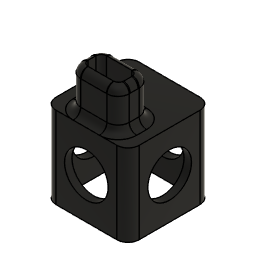
USB C Charger Protector v7 (Autodesk Fusion 360 design; units mm, degrees)
Autodesk Fusion 360 part; units mm, degrees
sketch "Sketch1" plane through (0, 0, 0) normal (0, 0, 1) x (1, 0, 0)
  line L0 (0, 0) -> (-27.6, 0)
  line L1 (-27.6, 0) -> (-27.6, 27.6)
  line L2 (-27.6, 27.6) -> (0, 27.6)
  line L3 (0, 27.6) -> (0, 0)
  line L4 (-27.6, 30.6) -> (-30.6, 30.6)
  line L5 (-30.6, 30.6) -> (3, 30.6)
  line L6 (3, 30.6) -> (3, -3)
  line L7 (3, -3) -> (-30.6, -3)
  line L8 (-30.6, -3) -> (-30.6, 30.6)
  dimension "d1" = 27.6
  dimension "d2" = 27.6
  dimension "d4" = 3
  dimension "d5" = 3
  dimension "d6" = 33.6
  dimension "d7" = 33.6
  constraint horizontal L0
  constraint vertical L1
  constraint horizontal L2
  constraint vertical L3
  constraint coincident L0.start L3.end
  constraint horizontal L5
  constraint vertical L6
  constraint horizontal L7
  constraint vertical L8
  measures "d1" distance of L0.start L0.end
  measures "d2" distance of L0.start L2.end
  measures "d4" distance of L1.end L4.start
  measures "d5" distance of L4.start L4.end
  measures "d6" distance of L4.end L5.end
  measures "d7" distance of L4.end L7.end
extrude "Extrude1" add sketch "Sketch1" along normal blind 30 makes body 1
sketch "Sketch2" plane through (0, 0, 30) normal (0, 0, 1) x (-1, 0, 0)
  line L0 (27.6, -27.6) -> (0, -27.6)
  line L1 (0, -27.6) -> (0, 0)
  line L2 (0, 0) -> (27.6, 0)
  line L3 (27.6, 0) -> (27.6, -27.6)
  line L4 (30.6, 3) -> (-3, 3)
  line L5 (-3, 3) -> (-3, -30.6)
  line L6 (-3, -30.6) -> (30.6, -30.6)
  line L7 (30.6, -30.6) -> (30.6, 3)
  line L8 (30.6, -30.6) -> (-3, -30.6)
  line L9 (-3, -30.6) -> (-3, 3)
  line L10 (-3, 3) -> (30.6, 3)
  line L11 (30.6, 3) -> (30.6, -30.6)
  constraint horizontal L8
  constraint vertical L9
  constraint horizontal L10
  constraint vertical L11
  constraint coincident L4.end L5.start
  constraint coincident L6.end L7.start
extrude "Extrude2" add sketch "Sketch2" along normal blind 3 contours L0 L1 L2 L3 | L4 L5 L6 L7 L8 L9 L10 L11 bodies 1
sketch "Sketch3" plane through (0, 0, 33) normal (0, 0, 1) x (-1, 0, 0)
  line L0 (30.6, 3) -> (-3, 3)
  line L1 (-3, 3) -> (-3, -30.6)
  line L2 (-3, -30.6) -> (30.6, -30.6)
  line L3 (30.6, -30.6) -> (30.6, 3)
  line L4 (18.9169, -2.769) -> (8.6831, -2.769)
  line L5 (6.5511, -4.901) -> (6.5511, -8.099)
  line L6 (8.6831, -10.231) -> (18.9169, -10.231)
  line L7 (21.0489, -8.099) -> (21.0489, -4.901)
  arc A0 (21.0489, -4.901) -> (18.9169, -2.769) centre (18.9169, -4.901) ccw
  arc A1 (18.9169, -10.231) -> (21.0489, -8.099) centre (18.9169, -8.099) ccw
  arc A2 (6.5511, -8.099) -> (8.6831, -10.231) centre (8.6831, -8.099) ccw
  arc A3 (8.6831, -2.769) -> (6.5511, -4.901) centre (8.6831, -4.901) ccw
  line L8 (19.1, -13) -> (8.5, -13)
  line L9 (4, -8.5) -> (4, -4.5)
  line L10 (8.5, 0) -> (19.1, 0)
  line L11 (23.6, -4.5) -> (23.6, -8.5)
  arc A4 (19.1, -13) -> (23.6, -8.5) centre (19.1, -8.5) ccw
  arc A5 (4, -8.5) -> (8.5, -13) centre (8.5, -8.5) ccw
  arc A6 (8.5, 0) -> (4, -4.5) centre (8.5, -4.5) ccw
  arc A7 (23.6, -4.5) -> (19.1, 0) centre (19.1, -4.5) ccw
  point P0 (21.0489, -2.769)
  point P1 (21.0489, -10.231)
  point P2 (23.6, -13)
  point P3 (4, 0)
  point P4 (13.8, -6.5)
  dimension "d62" = 4.5
  constraint vertical L5
  constraint vertical L7
  constraint coincident P0 L4
  constraint coincident P0 L7
  constraint coincident P1 L6
  constraint coincident P1 L7
  constraint horizontal L8
  constraint vertical L9
  constraint horizontal L10
  constraint vertical L11
  constraint tangent L8 A4
  constraint tangent L11 A4
  constraint tangent L8 A5
  constraint tangent L9 A5
  constraint equal A4 A5
  constraint tangent L9 A6
  constraint tangent L10 A6
  constraint equal A4 A6
  constraint tangent L10 A7
  constraint tangent L11 A7
  constraint equal A4 A7
  measures "d62" radius of A4
extrude "Extrude10" add sketch "Sketch3" along normal blind 16 contours L8 L9 L10 L11 A4 A5 A6 A7 bodies 1
fillet "Fillet1" radius 3 4 edges at (-27.6, 27.6, 15) (0, 27.6, 15) (0, 0, 15) (-27.6, 0, 15) on bodies 1
fillet "Fillet2" radius 4.5 4 edges at (3, -3, 16.5) (-30.6, -3, 16.5) (3, 30.6, 16.5) (-30.6, 30.6, 16.5) on bodies 1
sketch "Sketch4" plane through (-30.6, 0, 0) normal (-1, 0, 0) x (0, -1, 0)
  line L0 (-26.1, 33) -> (-26.1, 0)
  line L1 (-26.1, 0) -> (-1.5, 0)
  line L2 (-1.5, 0) -> (-1.5, 33)
  line L3 (-1.5, 33) -> (-26.1, 33)
  circle A0 centre (-13.8, 16.5) radius 8.8142
extrude "Extrude5" cut sketch "Sketch4" against normal blind 33.6 contours A0 bodies 1
sketch "Sketch5" plane through (0, -3, 0) normal (0, -1, 0) x (1, 0, 0)
  line L0 (-26.1, 33) -> (-26.1, 0)
  line L1 (-26.1, 0) -> (-1.5, 0)
  line L2 (-1.5, 0) -> (-1.5, 33)
  line L3 (-1.5, 33) -> (-26.1, 33)
  circle A0 centre (-13.8, 16.5) radius 8.8142
extrude "Extrude6" cut sketch "Sketch5" against normal blind 33.6 contours A0 bodies 1
sketch "Sketch6" plane through (0, 0, 0) normal (0, 0, 1) x (1, 0, 0)
  line L0 (-23.7662, 27.4159) -> (-3.7397, 27.4159)
  line L1 (-0.2397, 23.9159) -> (-0.2397, 3.7722)
  line L2 (-3.7397, 0.2722) -> (-23.7662, 0.2722)
  line L3 (-27.2662, 3.7722) -> (-27.2662, 23.9159)
  arc A0 (-3.7397, 0.2722) -> (-0.2397, 3.7722) centre (-3.7397, 3.7722) ccw
  arc A1 (-27.2662, 3.7722) -> (-23.7662, 0.2722) centre (-23.7662, 3.7722) ccw
  arc A2 (-23.7662, 27.4159) -> (-27.2662, 23.9159) centre (-23.7662, 23.9159) ccw
  arc A3 (-0.2397, 23.9159) -> (-3.7397, 27.4159) centre (-3.7397, 23.9159) ccw
  dimension "d36" = 3.5
  constraint horizontal L0
  constraint vertical L1
  constraint horizontal L2
  constraint vertical L3
  constraint tangent L1 A0
  constraint tangent L2 A0
  constraint tangent L2 A1
  constraint tangent L3 A1
  constraint equal A0 A1
  constraint tangent L0 A2
  constraint tangent L3 A2
  constraint equal A0 A2
  constraint tangent L0 A3
  constraint tangent L1 A3
  constraint equal A0 A3
  measures "d36" radius of A0
extrude "Extrude7" add sketch "Sketch6" along normal blind 29 separate body makes body 2
sketch "Sketch7" plane through (0, 0, 29) normal (0, 0, 1) x (-1, 0, 0)
  arc A0 (3.7397, -0.2722) -> (0.2397, -3.7722) centre (3.7397, -3.7722) ccw
  line L0 (0.2397, -3.7722) -> (0.2397, -23.9159)
  arc A1 (0.2397, -23.9159) -> (3.7397, -27.4159) centre (3.7397, -23.9159) ccw
  line L1 (3.7397, -27.4159) -> (23.7662, -27.4159)
  arc A2 (23.7662, -27.4159) -> (27.2662, -23.9159) centre (23.7662, -23.9159) ccw
  line L2 (27.2662, -23.9159) -> (27.2662, -3.7722)
  arc A3 (27.2662, -3.7722) -> (23.7662, -0.2722) centre (23.7662, -3.7722) ccw
  line L3 (23.7662, -0.2722) -> (3.7397, -0.2722)
  line L4 (18.3436, -8.89) -> (8.1175, -8.89)
  line L5 (8.1175, -4) -> (18.3287, -4)
  arc A4 (18.258, -8.89) -> (18.258, -4) centre (18.3436, -6.445) ccw
  arc A5 (8.1175, -4) -> (8.1175, -8.89) centre (8.1175, -6.445) ccw
  constraint horizontal L4
  constraint coincident L5 A4.end
  constraint coincident L4 A4.start
extrude "Extrude8" add sketch "Sketch7" along normal blind 19 contours L4 L5 A4 A5 bodies 2
sketch "Sketch8" plane through (0, 0, 48) normal (0, 0, 1) x (-1, 0, 0)
  arc A0 (18.258, -8.89) -> (18.258, -4) centre (18.3436, -6.445) ccw
  line L0 (18.258, -4) -> (8.1175, -4)
  arc A1 (8.1175, -4) -> (8.1175, -8.89) centre (8.1175, -6.445) ccw
  line L1 (8.1175, -8.89) -> (18.258, -8.89)
  circle A2 centre (13.1653, -6.445) radius 2.1966
extrude "Extrude9" add sketch "Sketch8" along normal blind 10 contours A2 bodies 2
sketch "Sketch9" plane through (0, 0, 58) normal (0, 0, 1) x (-1, 0, 0)
  circle A0 centre (13.1653, -6.445) radius 2.1966
  circle A1 centre (13.1653, -6.445) radius 1.665
  constraint concentric A0 A1
ref_plane "WorkPlane1" through (0, 6.445, 0) normal (0, 1, 0) x (0, 0, 1)
sketch "Sketch10" plane through (0, 6.445, 0) normal (0, 1, 0) x (1, 0, 0)
  spline S0 degree 5 poles (-13, -58) (-12.7715, -58.7573) (-12.3972, -60.2898) (-12.0836, -62.6418) (-12.1692, -65.8864) (-13.1619, -70.1327) (-15.0887, -74.5801) (-17.9612, -79.2311) (-21.716, -84.0721) (-26.2639, -89.0838) (-31.514, -94.2467) (-36.2176, -98.4854) (-40.0083, -101.7211) (-42.6503, -103.9029) (-44, -105) knots 0 0 0 0 0 0 0.1 0.2 0.3 0.4 0.5 0.6 0.7 0.8 0.9 1 1 1 1 1 1
  point P0 (-15, -74)
sweep "Sweep1" add profiles "Sketch9" path "Sketch10" along S0 section 1 contours A1 bodies 2
fillet "Fillet4" radius 3 16 edges at (-5.318, 11.682, 33) (-4, 6.5, 33) (-5.318, 1.318, 33) (-13.8, 0, 33) (-22.282, 1.318, 33) (-23.6, 6.5, 33) (-22.282, 11.682, 33) (-13.8, 13, 33) (-22.282, 1.318, 49) (-13.8, 0, 49) (-5.318, 1.318, 49) (-4, 6.5, 49) (-5.318, 11.682, 49) (-13.8, 13, 49) (-22.282, 11.682, 49) (-23.6, 6.5, 49) on bodies 1
extrude "Extrude11" cut 1 faces at (-15.5056, 7.7437, 33) along direction (0, 0, -1) blind 3 on bodies 1 bodies 1
hidden bodies 2
